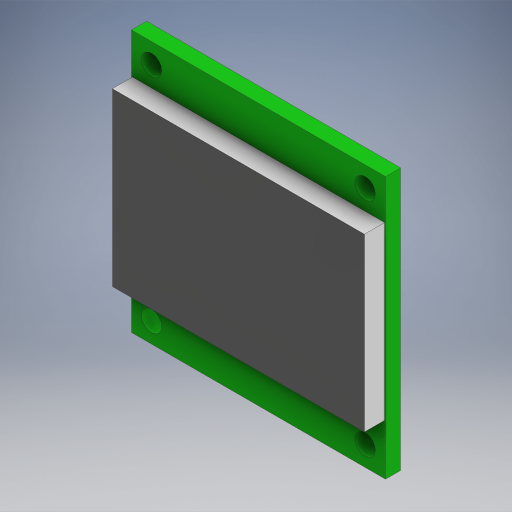
# Autodesk Inventor part: Дисплей
Saved by Autodesk Inventor 2023 (Build 270158000, 158)
## iProperties
Created: 2022-06-08
Part Number: Дисплей
Material: Типовые
Document SubType Name: Modeling
Designer: Admin
Density: 1 g/cm^3
Appearance: По умолчанию
Author: Admin
Autodesk Inventor part; units mm, degrees
ref_plane "YZ Plane" through (0, 0, 0) normal (1, 0, 0) x (0, 1, 0)
ref_plane "XZ Plane" through (0, 0, 0) normal (0, 1, 0) x (-1, 0, 0)
ref_plane "XY Plane" through (0, 0, 0) normal (0, 0, 1) x (1, 0, 0)
sketch "Эскиз1" plane through (0, 0, 0) normal (0, 0, 1) x (1, 0, 0)
  line L0 (-12.6, -13) -> (12.6, -13)
  line L1 (12.6, -13) -> (12.6, 13)
  line L2 (12.6, 13) -> (-12.6, 13)
  line L3 (-12.6, 13) -> (-12.6, -13)
  line L4 (-12.6, -13) -> (12.6, 13) construction
  line L5 (12.6, -13) -> (-12.6, 13) construction
  circle A0 centre (-10.6, 11) radius 1
  circle A1 centre (10.6, 11) radius 1
  circle A2 centre (10.6, -11) radius 1
  circle A3 centre (-10.6, -11) radius 1
  line L6 (12.5, -8) -> (-12.5, -8)
  line L7 (-12.5, -8) -> (-12.5, 9)
  line L8 (-12.5, 9) -> (12.5, 9)
  line L9 (12.5, 9) -> (12.5, -8)
  point P0 (0, 0)
  point P1 (0, -8)
  point P2 (0, 0)
  dimension "d0" = 25.2
  dimension "d1" = 26
  dimension "d4" = 2
  dimension "d13" = 2
  dimension "d14" = 2
  dimension "d15" = 2
  dimension "d16" = 2
  dimension "d17" = 2
  dimension "d18" = 2
  dimension "d19" = 2
  dimension "d20" = 2
  dimension "d25" = 25
  dimension "d26" = 17
  dimension "d29" = 5
  constraints: 20 end point, 4 centre point, 4 midpoint, 4 parallel, 3 equal radius, 2 horizontal, 2 perpendicular, 1 vertical alignment
  measures "d0" distance of L2.end L1.end
  measures "d1" distance of L1.end L0.end
  measures "d4" diameter of A0
  measures "d13" distance from line of L2 A1.centre
  measures "d14" distance from line of L1 A1.centre
  measures "d15" distance from line of L2 A0.centre
  measures "d16" distance from line of L3 A0.centre
  measures "d17" distance from line of L3 A3.centre
  measures "d18" distance from line of L0 A3.centre
  measures "d19" distance from line of L0 A2.centre
  measures "d20" distance from line of L1 A2.centre
  measures "d25" distance of L6.start L6.end
  measures "d26" distance of L6.end L7.end
  measures "d29" distance between parallel lines of L6 L0
extrude "Выдавливание1" add sketch "Эскиз1" against normal blind 1.5 contours L3 L2 L1 L0 | L6 L7 L8 L9
extrude "Выдавливание2" add sketch "Эскиз1" along normal blind 2 contours L6 L7 L8 L9
